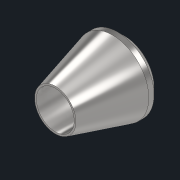
# Autodesk Inventor part: rod390_end_cap
Saved by Autodesk Inventor 2022 (Build 260153000, 153)
## iProperties
Created: 2024-03-31
Part Number: rod390_end_cap
Material: ステンレス鋼
Document SubType Name: Modeling
Designer: gisen
Mass: 187.662 g
Surface Area: 79.3058 cm^2
Volume: 23.4577 cm^3
Density: 8 g/cm^3
Appearance: 半つや出し
Author: gisen
Autodesk Inventor part; units mm, degrees
ref_plane "YZ Plane" through (0, 0, 0) normal (1, 0, 0) x (0, 1, 0)
ref_plane "XZ Plane" through (0, 0, 0) normal (0, 1, 0) x (-1, 0, 0)
ref_plane "XY Plane" through (0, 0, 0) normal (0, 0, 1) x (1, 0, 0)
sketch "スケッチ1" plane through (0, 0, 0) normal (1, 0, 0) x (0, 1, 0)
  line L0 (10.9, 20) -> (10.9, 0)
  line L1 (10.9, 0) -> (10, 0)
  line L2 (10, 0) -> (10, -20)
  line L3 (10, -20) -> (20.9, -20)
  line L4 (0, -28) -> (0, 28) projected
  line L5 (10.9, 20) -> (20.9, 20)
  line L6 (20.9, 20) -> (20.9, -20)
  point P0 (0, 0)
  dimension "d1" = 10
  dimension "d2" = 20
  dimension "d3" = 10.9
  dimension "d14" = 20.9
  dimension "d15" = 20
  constraints: 12 end point, 3 perpendicular, 2 vertical, 1 horizontal, 1 horizontal alignment
  measures "d1" distance from line of point (0, 0) L2
  measures "d2" distance of L1.end L2.end
  measures "d3" distance from line of point (0, 0) L0
  measures "d14" horizontal distance of point (0, 0) L3.end
  measures "d15" distance of L0.start L0.end
revolve "回転1" add sketch "スケッチ1" angle 360 about axis through (0, 0, -10) along (0, 0, 1)
thread "ねじ1" size "M20x2" class "6H" standard "ISO Metric profile" full length
chamfer "面取り1" distance 33 distance2 9 1 edges at (0, -20.9, 20) measured on face at (1.6818, 20.8322, -6.6667)
chamfer "面取り2" distance 4 angle 45 1 edges at (0, -20.9, -20)
